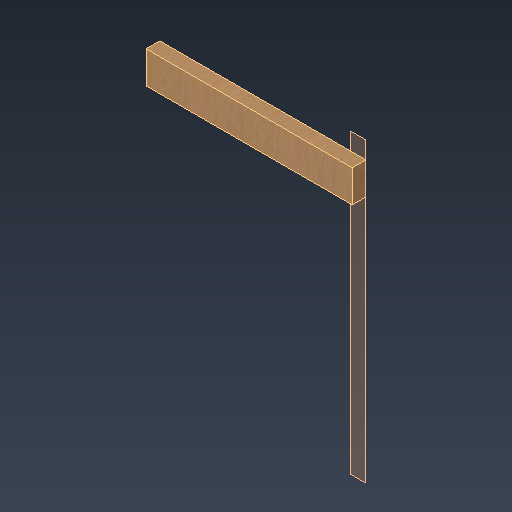
# Autodesk Inventor part: LSideBar
Saved by Autodesk Inventor 2021 (Build 250183000, 183)
## iProperties
Created: 2017-09-10
Part Number: LSideBar
Material: Wood
Document SubType Name: Modeling
Designer: jjsch
Density: 0.570257 g/cm^3
Appearance: Yellow Pine - Solid Natural Low Gloss
Mass: 1103.86 g
Surface Area: 1519.35 cm^2
Volume: 1935.72 cm^3
Author: jjsch
Autodesk Inventor part; units mm, degrees
ref_plane "YZ Plane" through (0, 0, 0) normal (1, 0, 0) x (0, 1, 0)
ref_plane "XZ Plane" through (0, 0, 0) normal (0, 1, 0) x (-1, 0, 0)
ref_plane "XY Plane" through (0, 0, 0) normal (0, 0, 1) x (1, 0, 0)
ref_plane "Work Plane1" through (-1377.161, -951.4221, 1748.0542) normal (0, 0, 1) x (1, 0, 0)
sketch "Sketch1" plane through (-1377.161, -951.4221, 1748.0542) normal (0, 0, 1) x (1, 0, 0)
  line L0 (21.0109, 364.1676) -> (-550.4891, 364.1676)
  line L1 (-550.4891, 364.1676) -> (-550.4891, 275.2676)
  line L2 (-550.4891, 275.2676) -> (21.0109, 275.2676)
  line L3 (21.0109, 275.2676) -> (21.0109, 364.1676)
  point P0 (1377.161, 951.4221)
  dimension "d0" = 571.5
  dimension "d1" = 88.9
  constraints: 8 end point, 2 parallel, 1 horizontal, 1 perpendicular
  measures "d0" distance of L2.end L1.end
  measures "d1" distance of L1.end L0.end
extrude "Extrusion1" add sketch "Sketch1" along normal blind 38.1
body "Solid1"
